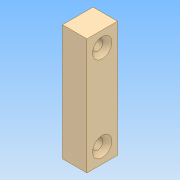
# Autodesk Inventor part: Top_End Sponge
Saved by Autodesk Inventor 2018.1 (Build 221171000, 171)
## iProperties
Created: 2019-03-22
Part Number: Top_End Sponge
Material: Rubber, Silicone
Document SubType Name: Modeling
Designer: James
Density: 1.25 g/cm^3
Appearance: Smooth - Off-White
Author: James
Autodesk Inventor part; units mm, degrees
ref_plane "YZ Plane" through (0, 0, 0) normal (1, 0, 0) x (0, 1, 0)
ref_plane "XZ Plane" through (0, 0, 0) normal (0, 1, 0) x (-1, 0, 0)
ref_plane "XY Plane" through (0, 0, 0) normal (0, 0, 1) x (1, 0, 0)
sketch "Sketch1" plane through (0, 0, 0) normal (0, 1, 0) x (-1, 0, 0)
  line L0 (0, 0) -> (8, 0)
  line L1 (8, 0) -> (8, -38)
  line L2 (8, -38) -> (0, -38)
  line L3 (0, -38) -> (0, 0)
  dimension "d0" = 38
  dimension "d1" = 8
  constraints: 8 end point, 2 parallel, 1 horizontal, 1 perpendicular
  measures "d0" distance of L0.end L1.end
  measures "d1" distance of L1.end L2.end
extrude "Extrusion1" add sketch "Sketch1" along normal blind 10
sketch "Sketch2" plane through (0, 0, 0) normal (1, 0, 0) x (0, 0, -1)
  line L0 (0, 0) -> (0, 10) projected
  line L1 (38, 0) -> (38, 10) projected
  point P0 (5, 5)
  point P1 (33, 5)
  point P2 (38, 5)
  dimension "d4" = 5
  dimension "d5" = 5
  constraints: 2 horizontal alignment, 1 midpoint
  measures "d4" distance from line of L0 point (5, 5)
  measures "d5" distance from line of L1 point (33, 5)
hole "Hole1" at (0, 5, -5) at (0, 5, -33) direction (-1, 0, 0) diameter 3.4 end through all countersink diameter 6.3 countersink angle 90 clearance for "Flat Head Machine Screw" size "M3" standard "Ansi Metric M Profile"
body "Solid1"
